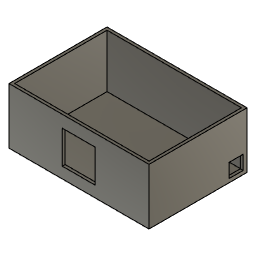
motionsensor-bottom (Autodesk Fusion 360 design; units mm, degrees)
Autodesk Fusion 360 part; units mm, degrees
note: some values were not read from the file. Set by a fixed rule: which face or edge a step refers to.
sketch "Sketch1" plane through (0, 0, 0) normal (0, 0, 1) x (1, 0, 0)
  line L0 (0, 0) -> (100, 0)
  line L1 (100, 0) -> (100, 70)
  line L2 (100, 70) -> (0, 70)
  line L3 (0, 70) -> (0, 0)
  dimension "d1" = 100
  dimension "d2" = 70
  constraint horizontal L0
  constraint vertical L1
  constraint horizontal L2
  constraint vertical L3
  constraint coincident L0.start L3.end
  measures "d1" distance of L0.start L0.end
  measures "d2" distance of L0.start L2.end
extrude "Extrude1" add sketch "Sketch1" along normal blind 40
sketch "Sketch2" plane through (0, 0, 0) normal (0, -1, 0) x (1, 0, 0)
  line L0 (0, 0) -> (100, 0)
  line L1 (100, 0) -> (100, 40)
  line L2 (100, 40) -> (0, 40)
  line L3 (0, 40) -> (0, 0)
  line L4 (38.0082, 31.4099, 5) -> (61.5082, 31.4099, 5)
  line L5 (61.5082, 31.4099, 5) -> (61.5082, 7.9099, 5)
  line L6 (61.5082, 7.9099, 5) -> (38.0082, 7.9099, 5)
  line L7 (38.0082, 7.9099, 5) -> (38.0082, 31.4099, 5)
  dimension "d5" = 23.5
  dimension "d6" = 23.5
extrude "Extrude2" cut sketch "Sketch2" against normal blind 10 contours L4 L5 L6 L7 in plane through (0, -5, 0) normal (0, -1, 0)
shell "Shell1" thickness 2 removed faces 1 at (33.3333, 46.6667, 40)
sketch "Sketch3" plane through (100, 0, 0) normal (1, 0, 0) x (0, 1, 0)
  line L0 (0, 0) -> (70, 0)
  line L1 (70, 0) -> (70, 40)
  line L2 (70, 40) -> (0, 40)
  line L3 (0, 40) -> (0, 0)
  line L4 (57.252, 12.6378) -> (67.252, 12.6378)
  line L5 (67.252, 12.6378) -> (67.252, 2.6378)
  line L6 (67.252, 2.6378) -> (57.252, 2.6378)
  line L7 (57.252, 2.6378) -> (57.252, 12.6378)
  constraint horizontal L4
  constraint vertical L5
  constraint horizontal L6
  constraint vertical L7
extrude "Extrude3" cut sketch "Sketch3" against normal blind 5 contours L4 L5 L6 L7
delete_face "DeleteFace1" 1 faces at (45.8415, 5, 23.5766)
delete_face "DeleteFace2" 1 faces at (45.1749, 3.6667, 33.4099)
